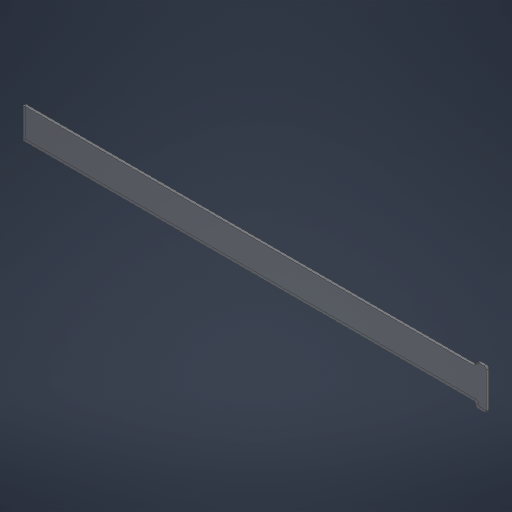
# Autodesk Inventor part: RACK_GUIDES
Saved by Autodesk Inventor 2026.2 (Build 302298010, 298A)
## iProperties
Created: 2026-04-01
Part Number: RACK_GUIDES
Material: Polycarbonate, PC 1000, Clear
Document SubType Name: Sheet Metal
Designer: 4aida
Density: 1.20131 g/cm^3
Sheet Metal Rule: Default
Appearance: Lexan (Clear)
Author: 4aida
Autodesk Inventor part; units mm, degrees
ref_plane "YZ Plane" through (0, 0, 0) normal (1, 0, 0) x (0, 1, 0)
ref_plane "XZ Plane" through (0, 0, 0) normal (0, 1, 0) x (-1, 0, 0)
ref_plane "XY Plane" through (0, 0, 0) normal (0, 0, 1) x (1, 0, 0)
sketch "Sketch1" plane through (0, 0, 0) normal (0, 0, 1) x (1, 0, 0)
  line L0 (279.4704, -19.05) -> (-282.4704, -19.05)
  line L1 (-282.4704, -19.05) -> (-282.4704, 19.05)
  line L2 (-282.4704, 19.05) -> (279.4704, 19.05)
  line L3 (282.4704, -19.05) -> (-282.4704, 19.05) construction
  line L4 (-282.4704, -19.05) -> (282.4704, 19.05) construction
  line L5 (292.1704, -25.05) -> (285.4704, -25.05)
  line L6 (285.4704, 25.05) -> (292.1704, 25.05)
  line L7 (295.1704, 22.05) -> (295.1704, -22.05)
  line L8 (295.1704, -25.05) -> (282.4704, 25.05) construction
  line L9 (282.4704, -25.05) -> (295.1704, 25.05) construction
  line L10 (282.4704, -22.05) -> (282.4704, -22.05)
  line L11 (282.4704, 22.05) -> (282.4704, 22.05)
  arc A0 (279.4704, 19.05) -> (282.4704, 22.05) centre (279.4704, 22.05) ccw
  arc A1 (285.4704, 25.05) -> (282.4704, 22.05) centre (285.4704, 22.05) ccw
  arc A2 (295.1704, 22.05) -> (292.1704, 25.05) centre (292.1704, 22.05) ccw
  arc A3 (292.1704, -25.05) -> (295.1704, -22.05) centre (292.1704, -22.05) ccw
  arc A4 (282.4704, -22.05) -> (285.4704, -25.05) centre (285.4704, -22.05) ccw
  arc A5 (282.4704, -22.05) -> (279.4704, -19.05) centre (279.4704, -22.05) ccw
  point P0 (0, 0)
  point P1 (288.8204, 0)
  point P2 (282.4704, 0)
  point P3 (295.1704, 0)
  dimension "d0" = 12.7
  dimension "d1" = 577.6407
  dimension "d2" = 6
  dimension "d3" = 38.1
  dimension "d4" = 3
  measures "d0" distance of L8.end L9.end
  measures "d1" distance between parallel lines of L7 L1
  measures "d2" distance between parallel lines of L2 L6
  measures "d3" distance between parallel lines of L2 L0
  measures "d4" radius of A0
extrude "Plate1" add sketch "Sketch1" along normal blind 3.175
equation "\"d5\" = Thickness"
equation "\"BendRadius\" = Thickness"
equation "\"BendReliefWidth\" = Thickness"
equation "\"BendReliefDepth\" = 0.5 * Thickness"
equation "\"CornerReliefSize\" = 4 * Thickness"
equation "\"MinimumRemnant\" = 2 * Thickness"
equation "\"TransitionRadius\" = BendRadius"
equation "\"JacobiRadiusSize\" = BendRadius"
equation "\"GapSize\" = Thickness"
equation "\"Thickness\" = 3.175"
body "Solid1"
